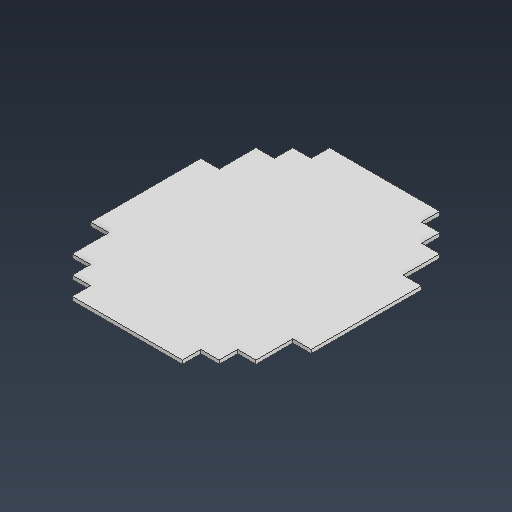
# Autodesk Inventor part: Shell
Saved by Autodesk Inventor 2025.3 (Build 293356000, 356)
## iProperties
Created: 2026-01-26
Part Number: Shell
Material: Generic
Document SubType Name: Modeling
Designer: tolga
Density: 1 g/cm^3
Appearance: Default
Author: tolga
Autodesk Inventor part; units mm, degrees
ref_plane "YZ Plane" through (0, 0, 0) normal (1, 0, 0) x (0, 1, 0)
ref_plane "XZ Plane" through (0, 0, 0) normal (0, 1, 0) x (-1, 0, 0)
ref_plane "XY Plane" through (0, 0, 0) normal (0, 0, 1) x (1, 0, 0)
sketch "Sketch1" plane through (0, 0, 0) normal (0, 1, 0) x (-1, 0, 0)
  line L0 (0, 0) -> (60, 0)
  line L1 (60, 0) -> (60, -10)
  line L2 (60, -10) -> (70, -10)
  line L3 (70, -10) -> (70, -20)
  line L4 (70, -20) -> (80, -20)
  line L5 (80, -20) -> (80, -40)
  line L6 (80, -40) -> (90, -40)
  line L7 (90, -40) -> (90, -100)
  line L8 (90, -70) -> (-110, -70) construction
  line L9 (30, 0) -> (30, -200) construction
  line L10 (0, -140) -> (60, -140)
  line L11 (60, -140) -> (60, -130)
  line L12 (60, -130) -> (70, -130)
  line L13 (70, -130) -> (70, -120)
  line L14 (70, -120) -> (80, -120)
  line L15 (80, -120) -> (80, -100)
  line L16 (80, -100) -> (90, -100)
  line L17 (0, 0) -> (0, -10)
  line L18 (0, -10) -> (-10, -10)
  line L19 (-10, -10) -> (-10, -20)
  line L20 (-10, -20) -> (-20, -20)
  line L21 (-20, -20) -> (-20, -40)
  line L22 (-20, -40) -> (-30, -40)
  line L23 (-30, -40) -> (-30, -100)
  line L24 (0, -140) -> (0, -130)
  line L25 (-10, -130) -> (-10, -120)
  line L26 (-10, -120) -> (-20, -120)
  line L27 (-20, -120) -> (-20, -100)
  line L28 (-20, -100) -> (-30, -100)
  line L29 (0, -130) -> (-10, -130)
  dimension "d0" = 10
  dimension "d1" = 60
  dimension "d2" = 10
  dimension "d3" = 10
  dimension "d4" = 20
  dimension "d5" = 60
  dimension "d6" = 10
  dimension "d7" = 10
  dimension "d8" = 200
  dimension "d9" = 200
  constraints: 60 end point, 19 symmetric about line, 6 perpendicular, 3 horizontal, 2 midpoint, 1 vertical
  measures "d0" distance of L0.end L1.end
  measures "d1" distance of L0.start L0.end
  measures "d2" distance of L2.end L3.end
  measures "d3" distance of L1.end L2.end
  measures "d4" distance of L4.end L5.end
  measures "d5" distance of L6.end L7.end
  measures "d6" distance of L3.end L4.end
  measures "d7" distance of L5.end L6.end
  measures "d8" distance of L8.start L8.end
  measures "d9" distance of L9.start L9.end
extrude "Extrusion1" add sketch "Sketch1" along normal blind 2
equation "\"d1\" = 6 * d0"
equation "\"d2\" = d0"
equation "\"d3\" = d0"
equation "\"d4\" = 2 * d0"
equation "\"d5\" = 6 * d0"
equation "\"d6\" = d0"
equation "\"d7\" = d0"
body "Solid1"
